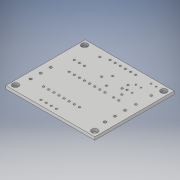
# Autodesk Inventor part: board
Saved by Autodesk Inventor 2019 (Build 230136000, 136)
## iProperties
Created: 2020-01-03
Part Number: board
Material: Типовые
Document SubType Name: Modeling
Designer: Петров Иван
Density: 1 g/cm^3
Appearance: По умолчанию
Author: Петров Иван
Autodesk Inventor part; units mm, degrees
ref_plane "YZ Plane" through (0, 0, 0) normal (1, 0, 0) x (0, 1, 0)
ref_plane "XZ Plane" through (0, 0, 0) normal (0, 1, 0) x (-1, 0, 0)
ref_plane "XY Plane" through (0, 0, 0) normal (0, 0, 1) x (1, 0, 0)
sketch "Эскиз2" plane through (0, 0, 0) normal (0, 1, 0) x (-1, 0, 0)
  arc A0 (55.499, 20.0698) -> (56.007, 20.0622) centre (55.753, 20.066) ccw
  arc A1 (56.134, 28.4442) -> (55.626, 28.4518) centre (55.88, 28.448) ccw
  line L0 (55.753, 20.066) -> (55.88, 28.448)
  arc A2 (68.834, 28.5703) -> (68.326, 28.5797) centre (68.58, 28.575) ccw
  line L1 (68.58, 28.575) -> (68.453, 21.717)
  arc A3 (68.199, 21.7217) -> (68.707, 21.7123) centre (68.453, 21.717) ccw
  arc A4 (70.993, 20.0622) -> (71.501, 20.0698) centre (71.247, 20.066) ccw
  arc A5 (71.374, 28.5788) -> (70.866, 28.5712) centre (71.12, 28.575) ccw
  line L2 (71.12, 28.575) -> (71.247, 20.066)
  line L3 (36.83, 0) -> (80.95, 0)
  line L4 (80.95, 0) -> (80.95, 39.36)
  line L5 (80.95, 39.36) -> (36.83, 39.36)
  line L6 (36.83, 39.36) -> (36.83, 0)
  circle A6 centre (39.37, 36.83) radius 1.5
  circle A7 centre (78.74, 36.83) radius 1.5
  circle A8 centre (78.74, 2.54) radius 1.5
  circle A9 centre (39.37, 2.54) radius 1.5
  line L7 (52.07, 5.588) -> (52.07, 0)
  arc A10 (53.34, 0.0318) -> (53.34, -0.0318) centre (53.34, 0) ccw
  line L8 (67.31, 5.588) -> (67.31, 0)
  arc A11 (67.2782, 0) -> (67.3418, 0) centre (67.31, 0) ccw
  arc A12 (67.3418, 5.588) -> (67.2782, 5.588) centre (67.31, 5.588) ccw
  arc A13 (52.07, 5.6197) -> (52.07, 5.5563) centre (52.07, 5.588) ccw
  arc A14 (52.0382, 0) -> (52.1018, 0) centre (52.07, 0) ccw
  arc A15 (52.1018, 5.588) -> (52.0382, 5.588) centre (52.07, 5.588) ccw
  line L9 (52.07, 5.588) -> (67.31, 5.588)
  arc A16 (67.31, 5.5563) -> (67.31, 5.6197) centre (67.31, 5.588) ccw
  arc A17 (66.04, -0.0318) -> (66.04, 0.0318) centre (66.04, 0) ccw
  line L10 (52.07, 0) -> (53.34, 0)
  arc A18 (53.34, -0.0318) -> (53.34, 0.0318) centre (53.34, 0) ccw
  arc A19 (52.07, 0.0318) -> (52.07, -0.0318) centre (52.07, 0) ccw
  line L11 (53.34, 0) -> (66.04, 0)
  arc A20 (53.34, 1.3017) -> (53.34, 1.2383) centre (53.34, 1.27) ccw
  arc A21 (66.04, 1.2383) -> (66.04, 1.3017) centre (66.04, 1.27) ccw
  line L12 (53.34, 1.27) -> (53.34, 0)
  arc A22 (53.3083, 0) -> (53.3718, 0) centre (53.3401, 0) ccw
  arc A23 (53.3718, 1.27) -> (53.3083, 1.27) centre (53.3401, 1.27) ccw
  line L13 (66.675, 3.81) -> (65.405, 3.81)
  arc A24 (65.405, 3.8608) -> (65.405, 3.7592) centre (65.405, 3.81) ccw
  arc A25 (66.675, 3.7592) -> (66.675, 3.8608) centre (66.675, 3.81) ccw
  arc A26 (66.0083, 0) -> (66.0718, 0) centre (66.0401, 0) ccw
  arc A27 (66.04, 0.0318) -> (66.04, -0.0318) centre (66.04, 0) ccw
  arc A28 (66.0718, 1.27) -> (66.0083, 1.27) centre (66.0401, 1.27) ccw
  line L14 (66.04, 1.27) -> (53.34, 1.27)
  line L15 (66.04, 0) -> (66.04, 1.27)
  arc A29 (67.31, -0.0318) -> (67.31, 0.0318) centre (67.31, 0) ccw
  line L16 (66.04, 0) -> (67.31, 0)
  line L17 (66.9798, 37.7698) -> (65.1002, 37.7698)
  line L18 (65.1002, 37.7698) -> (65.1002, 35.8902)
  line L19 (65.1002, 35.8902) -> (66.9798, 35.8902)
  line L20 (66.9798, 35.8902) -> (66.9798, 37.7698)
  line L21 (66.9798, 37.7698) -> (65.1002, 37.7698)
  line L22 (65.1002, 37.7698) -> (65.1002, 35.8902)
  line L23 (65.1002, 35.8902) -> (66.9798, 35.8902)
  line L24 (66.9798, 35.8902) -> (66.9798, 37.7698)
  arc A30 (63.5, 37.2999) -> (63.5, 36.3601) centre (63.5, 36.83) ccw
  arc A31 (63.5, 36.3601) -> (63.5, 37.2999) centre (63.5, 36.83) ccw
  arc A32 (63.5, 37.2999) -> (63.5, 36.3601) centre (63.5, 36.83) ccw
  arc A33 (63.5, 36.3601) -> (63.5, 37.2999) centre (63.5, 36.83) ccw
  arc A34 (60.96, 37.2999) -> (60.96, 36.3601) centre (60.96, 36.83) ccw
  arc A35 (60.96, 36.3601) -> (60.96, 37.2999) centre (60.96, 36.83) ccw
  arc A36 (60.96, 37.2999) -> (60.96, 36.3601) centre (60.96, 36.83) ccw
  arc A37 (60.96, 36.3601) -> (60.96, 37.2999) centre (60.96, 36.83) ccw
  arc A38 (58.42, 37.2999) -> (58.42, 36.3601) centre (58.42, 36.83) ccw
  arc A39 (58.42, 36.3601) -> (58.42, 37.2999) centre (58.42, 36.83) ccw
  arc A40 (58.42, 37.2999) -> (58.42, 36.3601) centre (58.42, 36.83) ccw
  arc A41 (58.42, 36.3601) -> (58.42, 37.2999) centre (58.42, 36.83) ccw
  arc A42 (66.04, 3.0099) -> (66.04, 2.0701) centre (66.04, 2.54) ccw
  arc A43 (66.04, 2.0701) -> (66.04, 3.0099) centre (66.04, 2.54) ccw
  arc A44 (66.04, 3.0099) -> (66.04, 2.0701) centre (66.04, 2.54) ccw
  arc A45 (66.04, 2.0701) -> (66.04, 3.0099) centre (66.04, 2.54) ccw
  arc A46 (63.5, 3.0099) -> (63.5, 2.0701) centre (63.5, 2.54) ccw
  arc A47 (63.5, 2.0701) -> (63.5, 3.0099) centre (63.5, 2.54) ccw
  arc A48 (63.5, 3.0099) -> (63.5, 2.0701) centre (63.5, 2.54) ccw
  arc A49 (63.5, 2.0701) -> (63.5, 3.0099) centre (63.5, 2.54) ccw
  arc A50 (60.96, 3.0099) -> (60.96, 2.0701) centre (60.96, 2.54) ccw
  arc A51 (60.96, 2.0701) -> (60.96, 3.0099) centre (60.96, 2.54) ccw
  arc A52 (60.96, 3.0099) -> (60.96, 2.0701) centre (60.96, 2.54) ccw
  arc A53 (60.96, 2.0701) -> (60.96, 3.0099) centre (60.96, 2.54) ccw
  arc A54 (58.42, 3.0099) -> (58.42, 2.0701) centre (58.42, 2.54) ccw
  arc A55 (58.42, 2.0701) -> (58.42, 3.0099) centre (58.42, 2.54) ccw
  arc A56 (58.42, 3.0099) -> (58.42, 2.0701) centre (58.42, 2.54) ccw
  arc A57 (58.42, 2.0701) -> (58.42, 3.0099) centre (58.42, 2.54) ccw
  arc A58 (55.88, 3.0099) -> (55.88, 2.0701) centre (55.88, 2.54) ccw
  arc A59 (55.88, 2.0701) -> (55.88, 3.0099) centre (55.88, 2.54) ccw
  arc A60 (55.88, 3.0099) -> (55.88, 2.0701) centre (55.88, 2.54) ccw
  arc A61 (55.88, 2.0701) -> (55.88, 3.0099) centre (55.88, 2.54) ccw
  arc A62 (53.34, 3.0099) -> (53.34, 2.0701) centre (53.34, 2.54) ccw
  arc A63 (53.34, 2.0701) -> (53.34, 3.0099) centre (53.34, 2.54) ccw
  arc A64 (53.34, 3.0099) -> (53.34, 2.0701) centre (53.34, 2.54) ccw
  arc A65 (53.34, 2.0701) -> (53.34, 3.0099) centre (53.34, 2.54) ccw
  line L25 (78.8035, 19.2405) -> (78.8035, 21.6535)
  line L26 (78.8035, 21.6535) -> (76.3905, 21.6535)
  line L27 (76.3905, 21.6535) -> (76.3905, 19.2405)
  line L28 (76.3905, 19.2405) -> (78.8035, 19.2405)
  line L29 (78.8035, 19.2405) -> (78.8035, 21.6535)
  line L30 (78.8035, 21.6535) -> (76.3905, 21.6535)
  line L31 (76.3905, 21.6535) -> (76.3905, 19.2405)
  line L32 (76.3905, 19.2405) -> (78.8035, 19.2405)
  arc A66 (78.2002, 25.447) -> (76.9938, 25.447) centre (77.597, 25.447) ccw
  arc A67 (76.9938, 25.447) -> (78.2002, 25.447) centre (77.597, 25.447) ccw
  arc A68 (78.2002, 25.447) -> (76.9938, 25.447) centre (77.597, 25.447) ccw
  arc A69 (76.9938, 25.447) -> (78.2002, 25.447) centre (77.597, 25.447) ccw
  arc A70 (78.2002, 30.447) -> (76.9938, 30.447) centre (77.597, 30.447) ccw
  arc A71 (76.9938, 30.447) -> (78.2002, 30.447) centre (77.597, 30.447) ccw
  arc A72 (78.2002, 30.447) -> (76.9938, 30.447) centre (77.597, 30.447) ccw
  arc A73 (76.9938, 30.447) -> (78.2002, 30.447) centre (77.597, 30.447) ccw
  line L33 (39.4335, 31.6865) -> (39.4335, 29.2735)
  line L34 (39.4335, 29.2735) -> (41.8465, 29.2735)
  line L35 (41.8465, 29.2735) -> (41.8465, 31.6865)
  line L36 (41.8465, 31.6865) -> (39.4335, 31.6865)
  line L37 (39.4335, 31.6865) -> (39.4335, 29.2735)
  line L38 (39.4335, 29.2735) -> (41.8465, 29.2735)
  line L39 (41.8465, 29.2735) -> (41.8465, 31.6865)
  line L40 (41.8465, 31.6865) -> (39.4335, 31.6865)
  arc A74 (40.0368, 25.48) -> (41.2433, 25.48) centre (40.64, 25.48) ccw
  arc A75 (41.2433, 25.48) -> (40.0368, 25.48) centre (40.64, 25.48) ccw
  arc A76 (40.0368, 25.48) -> (41.2433, 25.48) centre (40.64, 25.48) ccw
  arc A77 (41.2433, 25.48) -> (40.0368, 25.48) centre (40.64, 25.48) ccw
  arc A78 (40.0368, 20.48) -> (41.2433, 20.48) centre (40.64, 20.48) ccw
  arc A79 (41.2433, 20.48) -> (40.0368, 20.48) centre (40.64, 20.48) ccw
  arc A80 (40.0368, 20.48) -> (41.2433, 20.48) centre (40.64, 20.48) ccw
  arc A81 (41.2433, 20.48) -> (40.0368, 20.48) centre (40.64, 20.48) ccw
  line L41 (49.3522, 11.3128) -> (49.3522, 11.0392)
  line L42 (49.3522, 11.0392) -> (49.1588, 10.8458)
  line L43 (49.1588, 10.8458) -> (48.8852, 10.8458)
  line L44 (48.8852, 10.8458) -> (48.6918, 11.0392)
  line L45 (48.6918, 11.0392) -> (48.6918, 11.3128)
  line L46 (48.6918, 11.3128) -> (48.8852, 11.5062)
  line L47 (48.8852, 11.5062) -> (49.1588, 11.5062)
  line L48 (49.1588, 11.5062) -> (49.3522, 11.3128)
  line L49 (49.3522, 11.3128) -> (49.3522, 11.0392)
  line L50 (49.3522, 11.3128) -> (49.3522, 11.0392)
  line L51 (49.3522, 11.0392) -> (49.1588, 10.8458)
  line L52 (49.1588, 10.8458) -> (48.8852, 10.8458)
  line L53 (48.8852, 10.8458) -> (48.6918, 11.0392)
  line L54 (48.6918, 11.0392) -> (48.6918, 11.3128)
  line L55 (48.6918, 11.3128) -> (48.8852, 11.5062)
  line L56 (48.8852, 11.5062) -> (49.1588, 11.5062)
  line L57 (49.1588, 11.5062) -> (49.3522, 11.3128)
  line L58 (49.3522, 11.3128) -> (49.3522, 11.0392)
  line L59 (46.8122, 11.3128) -> (46.8122, 11.0392)
  line L60 (46.8122, 11.0392) -> (46.6188, 10.8458)
  line L61 (46.6188, 10.8458) -> (46.3452, 10.8458)
  line L62 (46.3452, 10.8458) -> (46.1518, 11.0392)
  line L63 (46.1518, 11.0392) -> (46.1518, 11.3128)
  line L64 (46.1518, 11.3128) -> (46.3452, 11.5062)
  line L65 (46.3452, 11.5062) -> (46.6188, 11.5062)
  line L66 (46.6188, 11.5062) -> (46.8122, 11.3128)
  line L67 (46.8122, 11.3128) -> (46.8122, 11.0392)
  line L68 (46.8122, 11.3128) -> (46.8122, 11.0392)
  line L69 (46.8122, 11.0392) -> (46.6188, 10.8458)
  line L70 (46.6188, 10.8458) -> (46.3452, 10.8458)
  line L71 (46.3452, 10.8458) -> (46.1518, 11.0392)
  line L72 (46.1518, 11.0392) -> (46.1518, 11.3128)
  line L73 (46.1518, 11.3128) -> (46.3452, 11.5062)
  line L74 (46.3452, 11.5062) -> (46.6188, 11.5062)
  line L75 (46.6188, 11.5062) -> (46.8122, 11.3128)
  line L76 (46.8122, 11.3128) -> (46.8122, 11.0392)
  line L77 (49.3522, 6.8678) -> (49.3522, 6.5942)
  line L78 (49.3522, 6.5942) -> (49.1588, 6.4008)
  line L79 (49.1588, 6.4008) -> (48.8852, 6.4008)
  line L80 (48.8852, 6.4008) -> (48.6918, 6.5942)
  line L81 (48.6918, 6.5942) -> (48.6918, 6.8678)
  line L82 (48.6918, 6.8678) -> (48.8852, 7.0612)
  line L83 (48.8852, 7.0612) -> (49.1588, 7.0612)
  line L84 (49.1588, 7.0612) -> (49.3522, 6.8678)
  line L85 (49.3522, 6.8678) -> (49.3522, 6.5942)
  line L86 (49.3522, 6.8678) -> (49.3522, 6.5942)
  line L87 (49.3522, 6.5942) -> (49.1588, 6.4008)
  line L88 (49.1588, 6.4008) -> (48.8852, 6.4008)
  line L89 (48.8852, 6.4008) -> (48.6918, 6.5942)
  line L90 (48.6918, 6.5942) -> (48.6918, 6.8678)
  line L91 (48.6918, 6.8678) -> (48.8852, 7.0612)
  line L92 (48.8852, 7.0612) -> (49.1588, 7.0612)
  line L93 (49.1588, 7.0612) -> (49.3522, 6.8678)
  line L94 (49.3522, 6.8678) -> (49.3522, 6.5942)
  line L95 (46.8122, 6.8678) -> (46.8122, 6.5942)
  line L96 (46.8122, 6.5942) -> (46.6188, 6.4008)
  line L97 (46.6188, 6.4008) -> (46.3452, 6.4008)
  line L98 (46.3452, 6.4008) -> (46.1518, 6.5942)
  line L99 (46.1518, 6.5942) -> (46.1518, 6.8678)
  line L100 (46.1518, 6.8678) -> (46.3452, 7.0612)
  line L101 (46.3452, 7.0612) -> (46.6188, 7.0612)
  line L102 (46.6188, 7.0612) -> (46.8122, 6.8678)
  line L103 (46.8122, 6.8678) -> (46.8122, 6.5942)
  line L104 (46.8122, 6.8678) -> (46.8122, 6.5942)
  line L105 (46.8122, 6.5942) -> (46.6188, 6.4008)
  line L106 (46.6188, 6.4008) -> (46.3452, 6.4008)
  line L107 (46.3452, 6.4008) -> (46.1518, 6.5942)
  line L108 (46.1518, 6.5942) -> (46.1518, 6.8678)
  line L109 (46.1518, 6.8678) -> (46.3452, 7.0612)
  line L110 (46.3452, 7.0612) -> (46.6188, 7.0612)
  line L111 (46.6188, 7.0612) -> (46.8122, 6.8678)
  line L112 (46.8122, 6.8678) -> (46.8122, 6.5942)
  line L113 (49.3522, 17.9168) -> (49.3522, 17.6432)
  line L114 (49.3522, 17.6432) -> (49.1588, 17.4498)
  line L115 (49.1588, 17.4498) -> (48.8852, 17.4498)
  line L116 (48.8852, 17.4498) -> (48.6918, 17.6432)
  line L117 (48.6918, 17.6432) -> (48.6918, 17.9168)
  line L118 (48.6918, 17.9168) -> (48.8852, 18.1102)
  line L119 (48.8852, 18.1102) -> (49.1588, 18.1102)
  line L120 (49.1588, 18.1102) -> (49.3522, 17.9168)
  line L121 (49.3522, 17.9168) -> (49.3522, 17.6432)
  line L122 (49.3522, 17.9168) -> (49.3522, 17.6432)
  line L123 (49.3522, 17.6432) -> (49.1588, 17.4498)
  line L124 (49.1588, 17.4498) -> (48.8852, 17.4498)
  line L125 (48.8852, 17.4498) -> (48.6918, 17.6432)
  line L126 (48.6918, 17.6432) -> (48.6918, 17.9168)
  line L127 (48.6918, 17.9168) -> (48.8852, 18.1102)
  line L128 (48.8852, 18.1102) -> (49.1588, 18.1102)
  line L129 (49.1588, 18.1102) -> (49.3522, 17.9168)
  line L130 (49.3522, 17.9168) -> (49.3522, 17.6432)
  line L131 (46.8122, 17.9168) -> (46.8122, 17.6432)
  line L132 (46.8122, 17.6432) -> (46.6188, 17.4498)
  line L133 (46.6188, 17.4498) -> (46.3452, 17.4498)
  line L134 (46.3452, 17.4498) -> (46.1518, 17.6432)
  line L135 (46.1518, 17.6432) -> (46.1518, 17.9168)
  line L136 (46.1518, 17.9168) -> (46.3452, 18.1102)
  line L137 (46.3452, 18.1102) -> (46.6188, 18.1102)
  line L138 (46.6188, 18.1102) -> (46.8122, 17.9168)
  line L139 (46.8122, 17.9168) -> (46.8122, 17.6432)
  line L140 (46.8122, 17.9168) -> (46.8122, 17.6432)
  line L141 (46.8122, 17.6432) -> (46.6188, 17.4498)
  line L142 (46.6188, 17.4498) -> (46.3452, 17.4498)
  line L143 (46.3452, 17.4498) -> (46.1518, 17.6432)
  line L144 (46.1518, 17.6432) -> (46.1518, 17.9168)
  line L145 (46.1518, 17.9168) -> (46.3452, 18.1102)
  line L146 (46.3452, 18.1102) -> (46.6188, 18.1102)
  line L147 (46.6188, 18.1102) -> (46.8122, 17.9168)
  line L148 (46.8122, 17.9168) -> (46.8122, 17.6432)
  line L149 (72.0598, 11.2932) -> (72.0598, 11.5668)
  line L150 (72.0598, 11.5668) -> (72.2532, 11.7602)
  line L151 (72.2532, 11.7602) -> (72.5268, 11.7602)
  line L152 (72.5268, 11.7602) -> (72.7202, 11.5668)
  line L153 (72.7202, 11.5668) -> (72.7202, 11.2932)
  line L154 (72.7202, 11.2932) -> (72.5268, 11.0998)
  line L155 (72.5268, 11.0998) -> (72.2532, 11.0998)
  line L156 (72.2532, 11.0998) -> (72.0598, 11.2932)
  line L157 (72.0598, 11.2932) -> (72.0598, 11.5668)
  line L158 (72.0598, 11.2932) -> (72.0598, 11.5668)
  line L159 (72.0598, 11.5668) -> (72.2532, 11.7602)
  line L160 (72.2532, 11.7602) -> (72.5268, 11.7602)
  line L161 (72.5268, 11.7602) -> (72.7202, 11.5668)
  line L162 (72.7202, 11.5668) -> (72.7202, 11.2932)
  line L163 (72.7202, 11.2932) -> (72.5268, 11.0998)
  line L164 (72.5268, 11.0998) -> (72.2532, 11.0998)
  line L165 (72.2532, 11.0998) -> (72.0598, 11.2932)
  line L166 (72.0598, 11.2932) -> (72.0598, 11.5668)
  line L167 (74.5998, 11.2932) -> (74.5998, 11.5668)
  line L168 (74.5998, 11.5668) -> (74.7932, 11.7602)
  line L169 (74.7932, 11.7602) -> (75.0668, 11.7602)
  line L170 (75.0668, 11.7602) -> (75.2602, 11.5668)
  line L171 (75.2602, 11.5668) -> (75.2602, 11.2932)
  line L172 (75.2602, 11.2932) -> (75.0668, 11.0998)
  line L173 (75.0668, 11.0998) -> (74.7932, 11.0998)
  line L174 (74.7932, 11.0998) -> (74.5998, 11.2932)
  line L175 (74.5998, 11.2932) -> (74.5998, 11.5668)
  line L176 (74.5998, 11.2932) -> (74.5998, 11.5668)
  line L177 (74.5998, 11.5668) -> (74.7932, 11.7602)
  line L178 (74.7932, 11.7602) -> (75.0668, 11.7602)
  line L179 (75.0668, 11.7602) -> (75.2602, 11.5668)
  line L180 (75.2602, 11.5668) -> (75.2602, 11.2932)
  line L181 (75.2602, 11.2932) -> (75.0668, 11.0998)
  line L182 (75.0668, 11.0998) -> (74.7932, 11.0998)
  line L183 (74.7932, 11.0998) -> (74.5998, 11.2932)
  line L184 (74.5998, 11.2932) -> (74.5998, 11.5668)
  line L185 (42.8498, 2.4032) -> (42.8498, 2.6768)
  line L186 (42.8498, 2.6768) -> (43.0432, 2.8702)
  line L187 (43.0432, 2.8702) -> (43.3168, 2.8702)
  line L188 (43.3168, 2.8702) -> (43.5102, 2.6768)
  line L189 (43.5102, 2.6768) -> (43.5102, 2.4032)
  line L190 (43.5102, 2.4032) -> (43.3168, 2.2098)
  line L191 (43.3168, 2.2098) -> (43.0432, 2.2098)
  line L192 (43.0432, 2.2098) -> (42.8498, 2.4032)
  line L193 (42.8498, 2.4032) -> (42.8498, 2.6768)
  line L194 (42.8498, 2.4032) -> (42.8498, 2.6768)
  line L195 (42.8498, 2.6768) -> (43.0432, 2.8702)
  line L196 (43.0432, 2.8702) -> (43.3168, 2.8702)
  line L197 (43.3168, 2.8702) -> (43.5102, 2.6768)
  line L198 (43.5102, 2.6768) -> (43.5102, 2.4032)
  line L199 (43.5102, 2.4032) -> (43.3168, 2.2098)
  line L200 (43.3168, 2.2098) -> (43.0432, 2.2098)
  line L201 (43.0432, 2.2098) -> (42.8498, 2.4032)
  line L202 (42.8498, 2.4032) -> (42.8498, 2.6768)
  line L203 (45.3898, 2.4032) -> (45.3898, 2.6768)
  line L204 (45.3898, 2.6768) -> (45.5832, 2.8702)
  line L205 (45.5832, 2.8702) -> (45.8568, 2.8702)
  line L206 (45.8568, 2.8702) -> (46.0502, 2.6768)
  line L207 (46.0502, 2.6768) -> (46.0502, 2.4032)
  line L208 (46.0502, 2.4032) -> (45.8568, 2.2098)
  line L209 (45.8568, 2.2098) -> (45.5832, 2.2098)
  line L210 (45.5832, 2.2098) -> (45.3898, 2.4032)
  line L211 (45.3898, 2.4032) -> (45.3898, 2.6768)
  line L212 (45.3898, 2.4032) -> (45.3898, 2.6768)
  line L213 (45.3898, 2.6768) -> (45.5832, 2.8702)
  line L214 (45.5832, 2.8702) -> (45.8568, 2.8702)
  line L215 (45.8568, 2.8702) -> (46.0502, 2.6768)
  line L216 (46.0502, 2.6768) -> (46.0502, 2.4032)
  line L217 (46.0502, 2.4032) -> (45.8568, 2.2098)
  line L218 (45.8568, 2.2098) -> (45.5832, 2.2098)
  line L219 (45.5832, 2.2098) -> (45.3898, 2.4032)
  line L220 (45.3898, 2.4032) -> (45.3898, 2.6768)
  line L221 (50.4698, 11.6742) -> (50.4698, 11.9478)
  line L222 (50.4698, 11.9478) -> (50.6632, 12.1412)
  line L223 (50.6632, 12.1412) -> (50.9368, 12.1412)
  line L224 (50.9368, 12.1412) -> (51.1302, 11.9478)
  line L225 (51.1302, 11.9478) -> (51.1302, 11.6742)
  line L226 (51.1302, 11.6742) -> (50.9368, 11.4808)
  line L227 (50.9368, 11.4808) -> (50.6632, 11.4808)
  line L228 (50.6632, 11.4808) -> (50.4698, 11.6742)
  line L229 (50.4698, 11.6742) -> (50.4698, 11.9478)
  line L230 (50.4698, 11.6742) -> (50.4698, 11.9478)
  line L231 (50.4698, 11.9478) -> (50.6632, 12.1412)
  line L232 (50.6632, 12.1412) -> (50.9368, 12.1412)
  line L233 (50.9368, 12.1412) -> (51.1302, 11.9478)
  line L234 (51.1302, 11.9478) -> (51.1302, 11.6742)
  line L235 (51.1302, 11.6742) -> (50.9368, 11.4808)
  line L236 (50.9368, 11.4808) -> (50.6632, 11.4808)
  line L237 (50.6632, 11.4808) -> (50.4698, 11.6742)
  line L238 (50.4698, 11.6742) -> (50.4698, 11.9478)
  line L239 (60.6298, 11.6742) -> (60.6298, 11.9478)
  line L240 (60.6298, 11.9478) -> (60.8232, 12.1412)
  line L241 (60.8232, 12.1412) -> (61.0968, 12.1412)
  line L242 (61.0968, 12.1412) -> (61.2902, 11.9478)
  line L243 (61.2902, 11.9478) -> (61.2902, 11.6742)
  line L244 (61.2902, 11.6742) -> (61.0968, 11.4808)
  line L245 (61.0968, 11.4808) -> (60.8232, 11.4808)
  line L246 (60.8232, 11.4808) -> (60.6298, 11.6742)
  line L247 (60.6298, 11.6742) -> (60.6298, 11.9478)
  line L248 (60.6298, 11.6742) -> (60.6298, 11.9478)
  line L249 (60.6298, 11.9478) -> (60.8232, 12.1412)
  line L250 (60.8232, 12.1412) -> (61.0968, 12.1412)
  line L251 (61.0968, 12.1412) -> (61.2902, 11.9478)
  line L252 (61.2902, 11.9478) -> (61.2902, 11.6742)
  line L253 (61.2902, 11.6742) -> (61.0968, 11.4808)
  line L254 (61.0968, 11.4808) -> (60.8232, 11.4808)
  line L255 (60.8232, 11.4808) -> (60.6298, 11.6742)
  line L256 (60.6298, 11.6742) -> (60.6298, 11.9478)
  line L257 (50.3174, 8.69) -> (50.3174, 9.09)
  line L258 (50.3174, 9.09) -> (50.6, 9.3726)
  line L259 (50.6, 9.3726) -> (51, 9.3726)
  line L260 (51, 9.3726) -> (51.2826, 9.09)
  line L261 (51.2826, 9.09) -> (51.2826, 8.69)
  line L262 (51.2826, 8.69) -> (51, 8.4074)
  line L263 (51, 8.4074) -> (50.6, 8.4074)
  line L264 (50.6, 8.4074) -> (50.3174, 8.69)
  line L265 (50.3174, 8.69) -> (50.3174, 9.09)
  line L266 (50.3174, 8.69) -> (50.3174, 9.09)
  line L267 (50.3174, 9.09) -> (50.6, 9.3726)
  line L268 (50.6, 9.3726) -> (51, 9.3726)
  line L269 (51, 9.3726) -> (51.2826, 9.09)
  line L270 (51.2826, 9.09) -> (51.2826, 8.69)
  line L271 (51.2826, 8.69) -> (51, 8.4074)
  line L272 (51, 8.4074) -> (50.6, 8.4074)
  line L273 (50.6, 8.4074) -> (50.3174, 8.69)
  line L274 (50.3174, 8.69) -> (50.3174, 9.09)
  line L275 (57.9374, 8.69) -> (57.9374, 9.09)
  line L276 (57.9374, 9.09) -> (58.22, 9.3726)
  line L277 (58.22, 9.3726) -> (58.62, 9.3726)
  line L278 (58.62, 9.3726) -> (58.9026, 9.09)
  line L279 (58.9026, 9.09) -> (58.9026, 8.69)
  line L280 (58.9026, 8.69) -> (58.62, 8.4074)
  line L281 (58.62, 8.4074) -> (58.22, 8.4074)
  line L282 (58.22, 8.4074) -> (57.9374, 8.69)
  line L283 (57.9374, 8.69) -> (57.9374, 9.09)
  line L284 (57.9374, 8.69) -> (57.9374, 9.09)
  line L285 (57.9374, 9.09) -> (58.22, 9.3726)
  line L286 (58.22, 9.3726) -> (58.62, 9.3726)
  line L287 (58.62, 9.3726) -> (58.9026, 9.09)
  line L288 (58.9026, 9.09) -> (58.9026, 8.69)
  line L289 (58.9026, 8.69) -> (58.62, 8.4074)
  line L290 (58.62, 8.4074) -> (58.22, 8.4074)
  line L291 (58.22, 8.4074) -> (57.9374, 8.69)
  line L292 (57.9374, 8.69) -> (57.9374, 9.09)
  line L293 (47.7774, 14.278) -> (47.7774, 14.678)
  line L294 (47.7774, 14.678) -> (48.06, 14.9606)
  line L295 (48.06, 14.9606) -> (48.46, 14.9606)
  line L296 (48.46, 14.9606) -> (48.7426, 14.678)
  line L297 (48.7426, 14.678) -> (48.7426, 14.278)
  line L298 (48.7426, 14.278) -> (48.46, 13.9954)
  line L299 (48.46, 13.9954) -> (48.06, 13.9954)
  line L300 (48.06, 13.9954) -> (47.7774, 14.278)
  line L301 (47.7774, 14.278) -> (47.7774, 14.678)
  line L302 (47.7774, 14.278) -> (47.7774, 14.678)
  line L303 (47.7774, 14.678) -> (48.06, 14.9606)
  line L304 (48.06, 14.9606) -> (48.46, 14.9606)
  line L305 (48.46, 14.9606) -> (48.7426, 14.678)
  line L306 (48.7426, 14.678) -> (48.7426, 14.278)
  line L307 (48.7426, 14.278) -> (48.46, 13.9954)
  line L308 (48.46, 13.9954) -> (48.06, 13.9954)
  line L309 (48.06, 13.9954) -> (47.7774, 14.278)
  line L310 (47.7774, 14.278) -> (47.7774, 14.678)
  line L311 (55.3974, 14.278) -> (55.3974, 14.678)
  line L312 (55.3974, 14.678) -> (55.68, 14.9606)
  line L313 (55.68, 14.9606) -> (56.08, 14.9606)
  line L314 (56.08, 14.9606) -> (56.3626, 14.678)
  line L315 (56.3626, 14.678) -> (56.3626, 14.278)
  line L316 (56.3626, 14.278) -> (56.08, 13.9954)
  line L317 (56.08, 13.9954) -> (55.68, 13.9954)
  line L318 (55.68, 13.9954) -> (55.3974, 14.278)
  line L319 (55.3974, 14.278) -> (55.3974, 14.678)
  line L320 (55.3974, 14.278) -> (55.3974, 14.678)
  line L321 (55.3974, 14.678) -> (55.68, 14.9606)
  line L322 (55.68, 14.9606) -> (56.08, 14.9606)
  line L323 (56.08, 14.9606) -> (56.3626, 14.678)
  line L324 (56.3626, 14.678) -> (56.3626, 14.278)
  line L325 (56.3626, 14.278) -> (56.08, 13.9954)
  line L326 (56.08, 13.9954) -> (55.68, 13.9954)
  line L327 (55.68, 13.9954) -> (55.3974, 14.278)
  line L328 (55.3974, 14.278) -> (55.3974, 14.678)
  line L329 (69.65, 11.9126) -> (70.05, 11.9126)
  line L330 (70.05, 11.9126) -> (70.3326, 11.63)
  line L331 (70.3326, 11.63) -> (70.3326, 11.23)
  line L332 (70.3326, 11.23) -> (70.05, 10.9474)
  line L333 (70.05, 10.9474) -> (69.65, 10.9474)
  line L334 (69.65, 10.9474) -> (69.3674, 11.23)
  line L335 (69.3674, 11.23) -> (69.3674, 11.63)
  line L336 (69.3674, 11.63) -> (69.65, 11.9126)
  line L337 (69.65, 11.9126) -> (70.05, 11.9126)
  line L338 (69.65, 11.9126) -> (70.05, 11.9126)
  line L339 (70.05, 11.9126) -> (70.3326, 11.63)
  line L340 (70.3326, 11.63) -> (70.3326, 11.23)
  line L341 (70.3326, 11.23) -> (70.05, 10.9474)
  line L342 (70.05, 10.9474) -> (69.65, 10.9474)
  line L343 (69.65, 10.9474) -> (69.3674, 11.23)
  line L344 (69.3674, 11.23) -> (69.3674, 11.63)
  line L345 (69.3674, 11.63) -> (69.65, 11.9126)
  line L346 (69.65, 11.9126) -> (70.05, 11.9126)
  line L347 (69.65, 4.2926) -> (70.05, 4.2926)
  line L348 (70.05, 4.2926) -> (70.3326, 4.01)
  line L349 (70.3326, 4.01) -> (70.3326, 3.61)
  line L350 (70.3326, 3.61) -> (70.05, 3.3274)
  line L351 (70.05, 3.3274) -> (69.65, 3.3274)
  line L352 (69.65, 3.3274) -> (69.3674, 3.61)
  line L353 (69.3674, 3.61) -> (69.3674, 4.01)
  line L354 (69.3674, 4.01) -> (69.65, 4.2926)
  line L355 (69.65, 4.2926) -> (70.05, 4.2926)
  line L356 (69.65, 4.2926) -> (70.05, 4.2926)
  line L357 (70.05, 4.2926) -> (70.3326, 4.01)
  line L358 (70.3326, 4.01) -> (70.3326, 3.61)
  line L359 (70.3326, 3.61) -> (70.05, 3.3274)
  line L360 (70.05, 3.3274) -> (69.65, 3.3274)
  line L361 (69.65, 3.3274) -> (69.3674, 3.61)
  line L362 (69.3674, 3.61) -> (69.3674, 4.01)
  line L363 (69.3674, 4.01) -> (69.65, 4.2926)
  line L364 (69.65, 4.2926) -> (70.05, 4.2926)
  line L365 (40.713, 7.1374) -> (40.313, 7.1374)
  line L366 (40.313, 7.1374) -> (40.0304, 7.42)
  line L367 (40.0304, 7.42) -> (40.0304, 7.82)
  line L368 (40.0304, 7.82) -> (40.313, 8.1026)
  line L369 (40.313, 8.1026) -> (40.713, 8.1026)
  line L370 (40.713, 8.1026) -> (40.9956, 7.82)
  line L371 (40.9956, 7.82) -> (40.9956, 7.42)
  line L372 (40.9956, 7.42) -> (40.713, 7.1374)
  line L373 (40.713, 7.1374) -> (40.313, 7.1374)
  line L374 (40.713, 7.1374) -> (40.313, 7.1374)
  line L375 (40.313, 7.1374) -> (40.0304, 7.42)
  line L376 (40.0304, 7.42) -> (40.0304, 7.82)
  line L377 (40.0304, 7.82) -> (40.313, 8.1026)
  line L378 (40.313, 8.1026) -> (40.713, 8.1026)
  line L379 (40.713, 8.1026) -> (40.9956, 7.82)
  line L380 (40.9956, 7.82) -> (40.9956, 7.42)
  line L381 (40.9956, 7.42) -> (40.713, 7.1374)
  line L382 (40.713, 7.1374) -> (40.313, 7.1374)
  line L383 (40.713, 14.7574) -> (40.313, 14.7574)
  line L384 (40.313, 14.7574) -> (40.0304, 15.04)
  line L385 (40.0304, 15.04) -> (40.0304, 15.44)
  line L386 (40.0304, 15.44) -> (40.313, 15.7226)
  line L387 (40.313, 15.7226) -> (40.713, 15.7226)
  line L388 (40.713, 15.7226) -> (40.9956, 15.44)
  line L389 (40.9956, 15.44) -> (40.9956, 15.04)
  line L390 (40.9956, 15.04) -> (40.713, 14.7574)
  line L391 (40.713, 14.7574) -> (40.313, 14.7574)
  line L392 (40.713, 14.7574) -> (40.313, 14.7574)
  line L393 (40.313, 14.7574) -> (40.0304, 15.04)
  line L394 (40.0304, 15.04) -> (40.0304, 15.44)
  line L395 (40.0304, 15.44) -> (40.313, 15.7226)
  line L396 (40.313, 15.7226) -> (40.713, 15.7226)
  line L397 (40.713, 15.7226) -> (40.9956, 15.44)
  line L398 (40.9956, 15.44) -> (40.9956, 15.04)
  line L399 (40.9956, 15.04) -> (40.713, 14.7574)
  line L400 (40.713, 14.7574) -> (40.313, 14.7574)
  line L401 (53.34, 17.126) -> (53.34, 18.434)
  arc A82 (53.667, 18.434) -> (53.013, 18.434) centre (53.34, 18.434) ccw
  arc A83 (53.013, 17.126) -> (53.667, 17.126) centre (53.34, 17.126) ccw
  line L402 (53.34, 17.126) -> (53.34, 18.434)
  arc A84 (53.667, 18.434) -> (53.013, 18.434) centre (53.34, 18.434) ccw
  arc A85 (53.013, 17.126) -> (53.667, 17.126) centre (53.34, 17.126) ccw
  line L403 (55.88, 17.126) -> (55.88, 18.434)
  arc A86 (56.207, 18.434) -> (55.553, 18.434) centre (55.88, 18.434) ccw
  arc A87 (55.553, 17.126) -> (56.207, 17.126) centre (55.88, 17.126) ccw
  line L404 (55.88, 17.126) -> (55.88, 18.434)
  arc A88 (56.207, 18.434) -> (55.553, 18.434) centre (55.88, 18.434) ccw
  arc A89 (55.553, 17.126) -> (56.207, 17.126) centre (55.88, 17.126) ccw
  line L405 (58.42, 17.126) -> (58.42, 18.434)
  arc A90 (58.747, 18.434) -> (58.093, 18.434) centre (58.42, 18.434) ccw
  arc A91 (58.093, 17.126) -> (58.747, 17.126) centre (58.42, 17.126) ccw
  line L406 (58.42, 17.126) -> (58.42, 18.434)
  arc A92 (58.747, 18.434) -> (58.093, 18.434) centre (58.42, 18.434) ccw
  arc A93 (58.093, 17.126) -> (58.747, 17.126) centre (58.42, 17.126) ccw
  line L407 (60.96, 17.126) -> (60.96, 18.434)
  arc A94 (61.287, 18.434) -> (60.633, 18.434) centre (60.96, 18.434) ccw
  arc A95 (60.633, 17.126) -> (61.287, 17.126) centre (60.96, 17.126) ccw
  line L408 (60.96, 17.126) -> (60.96, 18.434)
  arc A96 (61.287, 18.434) -> (60.633, 18.434) centre (60.96, 18.434) ccw
  arc A97 (60.633, 17.126) -> (61.287, 17.126) centre (60.96, 17.126) ccw
  line L409 (63.5, 17.126) -> (63.5, 18.434)
  arc A98 (63.827, 18.434) -> (63.173, 18.434) centre (63.5, 18.434) ccw
  arc A99 (63.173, 17.126) -> (63.827, 17.126) centre (63.5, 17.126) ccw
  line L410 (63.5, 17.126) -> (63.5, 18.434)
  arc A100 (63.827, 18.434) -> (63.173, 18.434) centre (63.5, 18.434) ccw
  arc A101 (63.173, 17.126) -> (63.827, 17.126) centre (63.5, 17.126) ccw
  line L411 (66.04, 17.126) -> (66.04, 18.434)
  arc A102 (66.367, 18.434) -> (65.713, 18.434) centre (66.04, 18.434) ccw
  arc A103 (65.713, 17.126) -> (66.367, 17.126) centre (66.04, 17.126) ccw
  line L412 (66.04, 17.126) -> (66.04, 18.434)
  arc A104 (66.367, 18.434) -> (65.713, 18.434) centre (66.04, 18.434) ccw
  arc A105 (65.713, 17.126) -> (66.367, 17.126) centre (66.04, 17.126) ccw
  line L413 (68.58, 17.126) -> (68.58, 18.434)
  arc A106 (68.907, 18.434) -> (68.253, 18.434) centre (68.58, 18.434) ccw
  arc A107 (68.253, 17.126) -> (68.907, 17.126) centre (68.58, 17.126) ccw
  line L414 (68.58, 17.126) -> (68.58, 18.434)
  arc A108 (68.907, 18.434) -> (68.253, 18.434) centre (68.58, 18.434) ccw
  arc A109 (68.253, 17.126) -> (68.907, 17.126) centre (68.58, 17.126) ccw
  line L415 (71.12, 17.126) -> (71.12, 18.434)
  arc A110 (71.447, 18.434) -> (70.793, 18.434) centre (71.12, 18.434) ccw
  arc A111 (70.793, 17.126) -> (71.447, 17.126) centre (71.12, 17.126) ccw
  line L416 (71.12, 17.126) -> (71.12, 18.434)
  arc A112 (71.447, 18.434) -> (70.793, 18.434) centre (71.12, 18.434) ccw
  arc A113 (70.793, 17.126) -> (71.447, 17.126) centre (71.12, 17.126) ccw
  line L417 (71.12, 29.826) -> (71.12, 31.134)
  arc A114 (71.447, 31.134) -> (70.793, 31.134) centre (71.12, 31.134) ccw
  arc A115 (70.793, 29.826) -> (71.447, 29.826) centre (71.12, 29.826) ccw
  line L418 (71.12, 29.826) -> (71.12, 31.134)
  arc A116 (71.447, 31.134) -> (70.793, 31.134) centre (71.12, 31.134) ccw
  arc A117 (70.793, 29.826) -> (71.447, 29.826) centre (71.12, 29.826) ccw
  line L419 (68.58, 29.826) -> (68.58, 31.134)
  arc A118 (68.907, 31.134) -> (68.253, 31.134) centre (68.58, 31.134) ccw
  arc A119 (68.253, 29.826) -> (68.907, 29.826) centre (68.58, 29.826) ccw
  line L420 (68.58, 29.826) -> (68.58, 31.134)
  arc A120 (68.907, 31.134) -> (68.253, 31.134) centre (68.58, 31.134) ccw
  arc A121 (68.253, 29.826) -> (68.907, 29.826) centre (68.58, 29.826) ccw
  line L421 (66.04, 29.826) -> (66.04, 31.134)
  arc A122 (66.367, 31.134) -> (65.713, 31.134) centre (66.04, 31.134) ccw
  arc A123 (65.713, 29.826) -> (66.367, 29.826) centre (66.04, 29.826) ccw
  line L422 (66.04, 29.826) -> (66.04, 31.134)
  arc A124 (66.367, 31.134) -> (65.713, 31.134) centre (66.04, 31.134) ccw
  arc A125 (65.713, 29.826) -> (66.367, 29.826) centre (66.04, 29.826) ccw
  line L423 (63.5, 29.826) -> (63.5, 31.134)
  arc A126 (63.827, 31.134) -> (63.173, 31.134) centre (63.5, 31.134) ccw
  arc A127 (63.173, 29.826) -> (63.827, 29.826) centre (63.5, 29.826) ccw
  line L424 (63.5, 29.826) -> (63.5, 31.134)
  arc A128 (63.827, 31.134) -> (63.173, 31.134) centre (63.5, 31.134) ccw
  arc A129 (63.173, 29.826) -> (63.827, 29.826) centre (63.5, 29.826) ccw
  line L425 (60.96, 29.826) -> (60.96, 31.134)
  arc A130 (61.287, 31.134) -> (60.633, 31.134) centre (60.96, 31.134) ccw
  arc A131 (60.633, 29.826) -> (61.287, 29.826) centre (60.96, 29.826) ccw
  line L426 (60.96, 29.826) -> (60.96, 31.134)
  arc A132 (61.287, 31.134) -> (60.633, 31.134) centre (60.96, 31.134) ccw
  arc A133 (60.633, 29.826) -> (61.287, 29.826) centre (60.96, 29.826) ccw
  line L427 (58.42, 29.826) -> (58.42, 31.134)
  arc A134 (58.747, 31.134) -> (58.093, 31.134) centre (58.42, 31.134) ccw
  arc A135 (58.093, 29.826) -> (58.747, 29.826) centre (58.42, 29.826) ccw
  line L428 (58.42, 29.826) -> (58.42, 31.134)
  arc A136 (58.747, 31.134) -> (58.093, 31.134) centre (58.42, 31.134) ccw
  arc A137 (58.093, 29.826) -> (58.747, 29.826) centre (58.42, 29.826) ccw
  line L429 (55.88, 29.826) -> (55.88, 31.134)
  arc A138 (56.207, 31.134) -> (55.553, 31.134) centre (55.88, 31.134) ccw
  arc A139 (55.553, 29.826) -> (56.207, 29.826) centre (55.88, 29.826) ccw
  line L430 (55.88, 29.826) -> (55.88, 31.134)
  arc A140 (56.207, 31.134) -> (55.553, 31.134) centre (55.88, 31.134) ccw
  arc A141 (55.553, 29.826) -> (56.207, 29.826) centre (55.88, 29.826) ccw
  line L431 (53.34, 29.826) -> (53.34, 31.134)
  arc A142 (53.667, 31.134) -> (53.013, 31.134) centre (53.34, 31.134) ccw
  arc A143 (53.013, 29.826) -> (53.667, 29.826) centre (53.34, 29.826) ccw
  line L432 (53.34, 29.826) -> (53.34, 31.134)
  arc A144 (53.667, 31.134) -> (53.013, 31.134) centre (53.34, 31.134) ccw
  arc A145 (53.013, 29.826) -> (53.667, 29.826) centre (53.34, 29.826) ccw
  arc A146 (68.453, 21.4154) -> (68.453, 22.0186) centre (68.453, 21.717) ccw
  arc A147 (68.453, 22.0186) -> (68.453, 21.4154) centre (68.453, 21.717) ccw
  arc A148 (68.453, 21.4154) -> (68.453, 22.0186) centre (68.453, 21.717) ccw
  arc A149 (68.453, 22.0186) -> (68.453, 21.4154) centre (68.453, 21.717) ccw
  arc A150 (68.58, 28.2734) -> (68.58, 28.8766) centre (68.58, 28.575) ccw
  arc A151 (68.58, 28.8766) -> (68.58, 28.2734) centre (68.58, 28.575) ccw
  arc A152 (68.58, 28.2734) -> (68.58, 28.8766) centre (68.58, 28.575) ccw
  arc A153 (68.58, 28.8766) -> (68.58, 28.2734) centre (68.58, 28.575) ccw
  arc A154 (55.753, 19.7644) -> (55.753, 20.3676) centre (55.753, 20.066) ccw
  arc A155 (55.753, 20.3676) -> (55.753, 19.7644) centre (55.753, 20.066) ccw
  arc A156 (55.753, 19.7644) -> (55.753, 20.3676) centre (55.753, 20.066) ccw
  arc A157 (55.753, 20.3676) -> (55.753, 19.7644) centre (55.753, 20.066) ccw
  arc A158 (71.247, 19.7644) -> (71.247, 20.3676) centre (71.247, 20.066) ccw
  arc A159 (71.247, 20.3676) -> (71.247, 19.7644) centre (71.247, 20.066) ccw
  arc A160 (71.247, 19.7644) -> (71.247, 20.3676) centre (71.247, 20.066) ccw
  arc A161 (71.247, 20.3676) -> (71.247, 19.7644) centre (71.247, 20.066) ccw
  arc A162 (55.88, 28.1464) -> (55.88, 28.7496) centre (55.88, 28.448) ccw
  arc A163 (55.88, 28.7496) -> (55.88, 28.1464) centre (55.88, 28.448) ccw
  arc A164 (55.88, 28.1464) -> (55.88, 28.7496) centre (55.88, 28.448) ccw
  arc A165 (55.88, 28.7496) -> (55.88, 28.1464) centre (55.88, 28.448) ccw
  arc A166 (71.12, 28.2734) -> (71.12, 28.8766) centre (71.12, 28.575) ccw
  arc A167 (71.12, 28.8766) -> (71.12, 28.2734) centre (71.12, 28.575) ccw
  arc A168 (71.12, 28.2734) -> (71.12, 28.8766) centre (71.12, 28.575) ccw
  arc A169 (71.12, 28.8766) -> (71.12, 28.2734) centre (71.12, 28.575) ccw
  circle A170 centre (40.64, 30.48) radius 0.6825
  circle A171 centre (77.597, 20.447) radius 0.6042
  circle A172 centre (66.04, 36.83) radius 0.47
  circle A173 centre (71.12, 30.48) radius 0.47
  circle A174 centre (71.12, 17.78) radius 0.47
  circle A175 centre (74.93, 11.43) radius 0.47
  circle A176 centre (72.39, 11.43) radius 0.47
  circle A177 centre (69.85, 11.43) radius 0.47
  circle A178 centre (69.85, 3.81) radius 0.47
  circle A179 centre (60.96, 11.811) radius 0.47
  circle A180 centre (58.42, 8.89) radius 0.47
  circle A181 centre (55.88, 14.478) radius 0.47
  circle A182 centre (48.26, 14.478) radius 0.47
  circle A183 centre (49.022, 17.78) radius 0.47
  circle A184 centre (46.482, 17.78) radius 0.47
  circle A185 centre (49.022, 11.176) radius 0.47
  circle A186 centre (50.8, 11.811) radius 0.47
  circle A187 centre (50.8, 8.89) radius 0.47
  circle A188 centre (49.022, 6.731) radius 0.3574
  circle A189 centre (46.482, 6.731) radius 0.3574
  circle A190 centre (46.482, 11.176) radius 0.3574
  circle A191 centre (40.513, 15.24) radius 0.5224
  circle A192 centre (40.513, 7.62) radius 0.5224
  circle A193 centre (43.18, 2.54) radius 0.3574
  circle A194 centre (45.72, 2.54) radius 0.3574
  circle A195 centre (68.58, 30.48) radius 0.47
  circle A196 centre (68.58, 17.78) radius 0.47
  circle A197 centre (66.04, 30.48) radius 0.47
  circle A198 centre (66.04, 17.78) radius 0.47
  circle A199 centre (63.5, 30.48) radius 0.47
  circle A200 centre (63.5, 17.78) radius 0.47
  circle A201 centre (60.96, 30.48) radius 0.47
  circle A202 centre (60.96, 17.78) radius 0.47
  circle A203 centre (58.42, 30.48) radius 0.47
  circle A204 centre (58.42, 17.78) radius 0.47
  circle A205 centre (55.88, 30.48) radius 0.47
  circle A206 centre (55.88, 17.78) radius 0.47
  circle A207 centre (53.34, 30.48) radius 0.47
  circle A208 centre (53.34, 17.78) radius 0.47
  line L433 (80.95, 39.36) -> (36.83, 39.36)
  line L434 (36.83, 39.36) -> (36.83, 0)
  line L435 (36.83, 0) -> (80.95, 0)
  line L436 (80.95, 0) -> (80.95, 39.36)
  circle A209 centre (40.64, 25.48) radius 0.6033
  circle A210 centre (40.64, 20.48) radius 0.6033
  circle A211 centre (77.597, 25.447) radius 0.6033
  circle A212 centre (77.597, 30.447) radius 0.6033
  circle A213 centre (63.5, 36.83) radius 0.4699
  circle A214 centre (60.96, 36.83) radius 0.4699
  circle A215 centre (58.42, 36.83) radius 0.4699
  circle A216 centre (63.5, 2.54) radius 0.4699
  circle A217 centre (66.04, 2.54) radius 0.4699
  circle A218 centre (60.96, 2.54) radius 0.4699
  circle A219 centre (58.42, 2.54) radius 0.4699
  circle A220 centre (55.88, 2.54) radius 0.4699
  circle A221 centre (53.34, 2.54) radius 0.4699
  point P0 (0, 0)
  point P1 (52.07, 14.478)
  point P2 (69.85, 7.62)
  point P3 (60.96, 25.4)
  point P4 (47.752, 11.176)
  point P5 (47.752, 6.731)
  point P6 (47.752, 17.78)
  point P7 (40.513, 11.43)
  point P8 (73.66, 11.43)
  point P9 (44.45, 2.54)
  point P10 (54.61, 8.89)
  point P11 (55.88, 11.811)
  dimension "d11" = 0.94
  dimension "d12" = 0.94
  dimension "d13" = 0.94
  dimension "d14" = 0.94
  dimension "d15" = 0.94
  dimension "d16" = 0.94
  dimension "d17" = 0.94
  dimension "d18" = 0.94
  dimension "d19" = 0.94
  dimension "d20" = 0.94
  dimension "d21" = 0.94
  dimension "d22" = 0.94
  dimension "d23" = 0.94
  dimension "d24" = 0.94
  dimension "d25" = 0.94
  dimension "d26" = 0.94
  dimension "d29" = 2.54
  constraints: 874 end point, 332 point on circle, 217 centre point, 16 coincident, 13 concentric, 2 horizontal, 2 midpoint, 2 parallel, 1 perpendicular, 43 other
  measures "d11" diameter of A172
  measures "d12" diameter of A173
  measures "d13" diameter of A174
  measures "d14" diameter of A175
  measures "d15" diameter of A176
  measures "d16" diameter of A177
  measures "d17" diameter of A178
  measures "d18" diameter of A179
  measures "d19" diameter of A180
  measures "d20" diameter of A181
  measures "d21" diameter of A182
  measures "d22" diameter of A183
  measures "d23" diameter of A184
  measures "d24" diameter of A185
  measures "d25" diameter of A186
  measures "d26" diameter of A187
  measures "d29" distance of A173.centre A195.centre
extrude "Выдавливание2" add sketch "Эскиз2" along normal blind 1.5 contours L6 L5 L4 L3 A29 L8 A16 A12 L9 A15 A13 L7 A19 | A19 L7 L3 | L7 L9 L8 L3 A17 L15 A21 A28 L14 A23 A20 L12 A10 | A13 A15 L9 L7 | A10 L12 L3 | L3 L8 A29 | L12 A18 L3 | L12 L14 L15 A27 L3 A18 | A20 A23 L14 L12 | A12 A16 L8 L9 | A27 L15 L3 | L3 L15 A17 | L15 L14 A28 A21 | L20 L19 L18 L17 | L28 L27 L26 L25 | L36 L35 L34 L33 | L257 L258 L259 L260 L261 L262 L263 L264 | L275 L276 L277 L278 L279 L280 L281 L282 | L293 L294 L295 L296 L297 L298 L299 L300 | L311 L312 L313 L314 L315 L316 L317 L318 | L329 L330 L331 L332 L333 L334 L335 L336 | L347 L348 L349 L350 L351 L352 L353 L354 | A147 A146 | A151 A150 | A155 A154 | A159 A158 | A163 A162 | A167 A166
